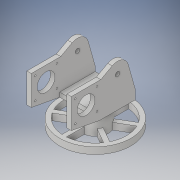
# Autodesk Inventor part: shoulder
Saved by Autodesk Inventor 2019 (Build 230136000, 136)
## iProperties
Created: 2019-05-02
Part Number: shoulder
Material: Generic
Document SubType Name: Modeling
Designer: Nathan
Density: 1 g/cm^3
Appearance: Default
Author: Nathan
Autodesk Inventor part; units mm, degrees
ref_plane "YZ Plane" through (0, 0, 0) normal (1, 0, 0) x (0, 1, 0)
ref_plane "XZ Plane" through (0, 0, 0) normal (0, 1, 0) x (-1, 0, 0)
ref_plane "XY Plane" through (0, 0, 0) normal (0, 0, 1) x (1, 0, 0)
sketch "Sketch1" plane through (0, 0, 0) normal (0, 1, 0) x (-1, 0, 0)
  circle A0 centre (0, 0) radius 50.8
  line L0 (3.175, -18.7836) -> (3.175, -44.3365)
  line L1 (-3.175, -18.7836) -> (-3.175, -44.3365)
  line L2 (0, -71.12) -> (0, 71.12) construction
  line L3 (17.8545, -6.6421) -> (39.984, -19.4186)
  line L4 (14.6795, -12.1414) -> (36.809, -24.9179)
  line L5 (14.6795, 12.1414) -> (36.809, 24.9179)
  line L6 (17.8545, 6.6421) -> (39.984, 19.4186)
  line L7 (-3.175, 18.7836) -> (-3.175, 44.3365)
  line L8 (3.175, 18.7836) -> (3.175, 44.3365)
  line L9 (-17.8545, 6.6421) -> (-39.984, 19.4186)
  line L10 (-14.6795, 12.1414) -> (-36.809, 24.9179)
  line L11 (-14.6795, -12.1414) -> (-36.809, -24.9179)
  line L12 (-17.8545, -6.6421) -> (-39.984, -19.4186)
  arc A1 (-14.6795, -12.1414) -> (-3.175, -18.7836) centre (0, 0) ccw
  arc A2 (-36.809, -24.9179) -> (-3.175, -44.3365) centre (0, 0) ccw
  arc A3 (-39.984, 19.4186) -> (-39.984, -19.4186) centre (0, 0) ccw
  arc A4 (-17.8545, 6.6421) -> (-17.8545, -6.6421) centre (0, 0) ccw
  arc A5 (-3.175, 18.7836) -> (-14.6795, 12.1414) centre (0, 0) ccw
  arc A6 (-3.175, 44.3365) -> (-36.809, 24.9179) centre (0, 0) ccw
  arc A7 (36.809, 24.9179) -> (3.175, 44.3365) centre (0, 0) ccw
  arc A8 (14.6795, 12.1414) -> (3.175, 18.7836) centre (0, 0) ccw
  arc A9 (3.175, -18.7836) -> (14.6795, -12.1414) centre (0, 0) ccw
  arc A10 (17.8545, -6.6421) -> (17.8545, 6.6421) centre (0, 0) ccw
  arc A11 (3.175, -44.3365) -> (36.809, -24.9179) centre (0, 0) ccw
  arc A12 (39.984, -19.4186) -> (39.984, 19.4186) centre (0, 0) ccw
  dimension "d6" = 360
  dimension "d0" = 101.6
  dimension "d3" = 6.35
  dimension "d8" = 19.05
  dimension "d9" = 6.35
  constraints: 24 end point, 24 point on circle, 13 centre point, 2 coincident, 2 parallel, 38 other
  measures "d0" diameter of A0
  measures "d3" distance between parallel lines of L1 L0
  measures "d8" radius of A9
  measures "d9" radial gap between concentric circles of A0 A3
extrude "Extrusion1" add sketch "Sketch1" along normal blind 9.525
sketch "Sketch2" plane through (0, 9.525, 0) normal (0, 1, 0) x (1, 0, 0)
  arc A0 (-17.8545, 6.6421) -> (-17.8545, -6.6421) centre (0, 0) ccw projected
  circle A1 centre (0, 0) radius 19.05
  constraints: 1 centre point, 1 coincident, 1 concentric
extrude "Extrusion2" add sketch "Sketch2" along normal blind 25.4
sketch "Sketch3" plane through (0, 34.925, 0) normal (0, 1, 0) x (1, 0, 0)
  line L0 (-31.75, 25.4) -> (31.75, 25.4)
  line L1 (31.75, 25.4) -> (31.75, -25.4)
  line L2 (31.75, -25.4) -> (-31.75, -25.4)
  line L3 (-31.75, -25.4) -> (-31.75, 25.4)
  point P0 (0, 0)
  point P1 (31.75, 0)
  point P2 (0, 25.4)
  dimension "d14" = 63.5
  dimension "d15" = 50.8
  constraints: 8 end point, 2 midpoint, 2 parallel, 1 horizontal, 1 horizontal alignment, 1 perpendicular, 1 vertical alignment
  measures "d14" distance of L0.start L0.end
  measures "d15" distance of L0.end L1.end
extrude "Extrusion3" add sketch "Sketch3" along normal blind 6.35
sketch "Sketch4" plane through (-31.75, 34.925, -25.4) normal (-1, 0, 0) x (0, 0, 1)
  line L0 (0, 6.35) -> (50.8, 6.35) projected
  circle A0 centre (25.4, 44.45) radius 31.75 construction
  circle A1 centre (70.3013, 28.575) radius 15.875 construction
  line L1 (49.3013, 49.575) -> (91.3013, 49.575)
  line L2 (91.3013, 49.575) -> (91.3013, 7.575)
  line L3 (91.3013, 7.575) -> (49.3013, 7.575) construction
  line L4 (49.3013, 7.575) -> (49.3013, 49.575) construction
  line L5 (85.8013, 44.075) -> (54.8013, 44.075) construction
  line L6 (54.8013, 44.075) -> (54.8013, 13.075) construction
  line L7 (54.8013, 13.075) -> (85.8013, 13.075) construction
  line L8 (85.8013, 13.075) -> (85.8013, 44.075) construction
  circle A2 centre (70.3013, 28.575) radius 12.7
  circle A3 centre (54.8013, 44.075) radius 1.25
  circle A4 centre (85.8013, 44.075) radius 1.25
  circle A5 centre (85.8013, 13.075) radius 1.25
  circle A6 centre (54.8013, 13.075) radius 1.25
  circle A7 centre (25.4, 44.45) radius 3.175
  arc A8 (32.9496, 58.4149) -> (10.1156, 48.74) centre (25.4, 44.45) ccw
  line L9 (0, 6.35) -> (0, 12.7)
  line L10 (0, 12.7) -> (10.1156, 48.74)
  line L11 (32.9496, 58.4149) -> (49.3013, 49.575)
  line L12 (50.8, 0) -> (91.3013, 7.575)
  line L13 (50.8, 0) -> (50.8, 6.35) projected
  point P0 (25.4, -34.925)
  point P1 (25.4, 6.35)
  point P2 (25.4, 12.7)
  point P3 (70.3013, 12.7)
  point P4 (91.3013, 28.575)
  point P5 (70.3013, 49.575)
  dimension "d18" = 63.5
  dimension "d19" = 31.75
  dimension "d20" = 38.1
  dimension "d21" = 42
  dimension "d22" = 42
  dimension "d23" = 5.5
  dimension "d24" = 25.4
  dimension "d25" = 2.5
  dimension "d26" = 6.35
  dimension "d27" = 12.7
  dimension "d28" = 6.35
  constraints: 24 end point, 7 centre point, 6 coincident, 6 vertical alignment, 4 parallel, 3 equal radius, 3 midpoint, 2 horizontal alignment, 2 perpendicular, 2 point on circle, 2 tangent, 1 horizontal, 1 vertical, 7 other
  measures "d20" distance of point (25.4, 6.35) point (25.4, 44.45)
  measures "d21" distance of L2.end L3.end
  measures "d22" distance of L1.end L2.end
  measures "d23" distance between parallel lines of L1 L5
  measures "d24" diameter of A2
  measures "d25" diameter of A3
  measures "d26" diameter of A7
  measures "d27" radial gap between concentric circles of A7 A8
  measures "d28" distance of L0.start L9.end
extrude "Extrusion4" add sketch "Sketch4" against normal blind 6.35
mirror "Mirror1" about plane through (0, 0, 0) normal (1, 0, 0) of "Extrusion4"
equation "\"d0\" = turntable_diameter"
equation "\"d3\" = turntable_spur_thickness"
equation "\"d8\" = 0.5 * spine_diameter"
equation "\"d9\" = turntable_spur_thickness"
equation "\"d10\" = turntable_thickness"
equation "\"d12\" = shoulder_height_offset"
equation "\"d14\" = shoulder_width"
equation "\"d15\" = shoulder_length"
equation "\"d16\" = shoulder_wall_thickness"
equation "\"d18\" = arm_proximal_gear_diameter"
equation "\"d19\" = shoulder_motor_gear_diameter"
equation "\"d20\" = 0.5 * arm_proximal_gear_diameter + shoulder_wall_thickness"
equation "\"d28\" = shoulder_wall_thickness"
equation "\"d29\" = shoulder_wall_thickness"
equation "\"turntable_diameter\" = 101.6"
equation "\"turntable_thickness\" = 9.525"
equation "\"shoulder_height_offset\" = 25.4"
equation "\"spine_diameter\" = 38.1"
equation "\"shoulder_width\" = 63.5"
equation "\"shoulder_wall_thickness\" = 6.35"
equation "\"shoulder_length\" = 50.8"
equation "\"arm_proximal_gear_diameter\" = 63.5"
equation "\"shoulder_motor_gear_diameter\" = 31.75"
equation "\"arm_proximal_gear_thickness\" = 9.525"
equation "\"arm_proximal_length\" = 177.8"
equation "\"arm_proximal_width\" = 12.7"
equation "\"turntable_spur_thickness\" = 6.35"
equation "\"base_height\" = 12.7"
equation "\"base_width\" = 165.1"
equation "\"base_length\" = 127"
equation "\"retention_poles_diameter\" = 6.35"
equation "\"turntable_bed_depth\" = 6.35"
equation "\"waist_cutout_overlap\" = 6.35"
equation "\"waist_motor_cutout_diameter\" = 50.8"
equation "\"base_motor_standoff_thickness\" = 3.175"
equation "\"base_motor_standoff_length\" = 63.5"
equation "\"base_motor_standoff_height\" = 12.7"
equation "\"base_motor_standoff_offset\" = 0"
body "Solid1"
